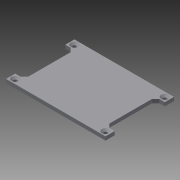
# Autodesk Inventor part: main body cover
Saved by Autodesk Inventor 2015 (Build 190159000, 159)
## iProperties
Created: 2019-05-11
Part Number: main body cover
Material: Generic
Document SubType Name: Modeling
Designer: Toby
Density: 1 g/cm^3
Appearance: Default
Author: Toby
Autodesk Inventor part; units mm, degrees
ref_plane "YZ Plane" through (0, 0, 0) normal (1, 0, 0) x (0, 1, 0)
ref_plane "XZ Plane" through (0, 0, 0) normal (0, 1, 0) x (-1, 0, 0)
ref_plane "XY Plane" through (0, 0, 0) normal (0, 0, 1) x (1, 0, 0)
sketch "Sketch1" plane through (0, 0, 0) normal (0, 0, 1) x (1, 0, 0)
  line L0 (-30.3644, 10.862) -> (24.0356, 10.862)
  line L1 (24.0356, 10.862) -> (24.0356, -26.538)
  line L2 (24.0356, -26.538) -> (-30.3644, -26.538)
  line L3 (-30.3644, -26.538) -> (-30.3644, 10.862)
  point P0 (0, 0)
  dimension "d0" = 54.4
  dimension "d1" = 37.4
  constraints: 8 end point, 2 parallel, 1 horizontal, 1 perpendicular
  measures "d0" distance of L0.start L0.end
  measures "d1" distance of L2.end L0.start
extrude "Extrusion1" add sketch "Sketch1" along normal blind 2
sketch "Sketch2" plane through (0, 0, 2) normal (0, 0, 1) x (1, 0, 0)
  line L0 (-30.3644, 10.862) -> (24.0356, 10.862) projected
  line L1 (-30.3644, 10.862) -> (-30.3644, -26.538) projected
  line L2 (-30.3644, -26.538) -> (24.0356, -26.538) projected
  line L3 (24.0356, -26.538) -> (24.0356, 10.862) projected
  point P0 (0, 0)
  point P1 (-27.8644, 8.362)
  point P2 (21.5356, -24.038)
  point P3 (21.5356, 8.362)
  point P4 (-27.8644, -24.038)
  dimension "d4" = 2.5
  dimension "d5" = 2.5
  dimension "d6" = 2.5
  dimension "d7" = 2.5
  measures "d4" distance from line of L0 point (-27.864, 8.362)
  measures "d5" distance from line of L1 point (-27.864, 8.362)
  measures "d6" distance from line of L2 point (21.536, -24.038)
  measures "d7" distance from line of L3 point (21.536, -24.038)
hole "Hole1" at (-27.8644, 8.362, 2) at (21.5356, -24.038, 2) at (21.5356, 8.362, 2) at (-27.8644, -24.038, 2) direction (0, 0, -1) diameter 2 depth 8 tip angle 118 countersink diameter 4 countersink angle 90
sketch "Sketch3" plane through (0, 0, 2) normal (0, 0, 1) x (1, 0, 0)
  line L0 (-30.3644, -26.538) -> (-30.3644, 10.862) projected
  line L1 (-30.3644, 5.862) -> (-25.3644, 5.862)
  line L2 (-25.3644, 5.862) -> (-25.3644, -21.538)
  line L3 (-25.3644, -21.538) -> (-30.3644, -21.538)
  line L4 (-30.3644, -21.538) -> (-30.3644, 5.862)
  line L5 (24.0356, 10.862) -> (24.0356, -26.538) projected
  line L6 (24.0356, 5.862) -> (19.0356, 5.862)
  line L7 (19.0356, 5.862) -> (19.0356, -21.538)
  line L8 (19.0356, -21.538) -> (24.0356, -21.538)
  line L9 (24.0356, -21.538) -> (24.0356, 5.862)
  line L10 (24.0356, 10.862) -> (-30.3644, 10.862) projected
  line L11 (-30.3644, -26.538) -> (24.0356, -26.538) projected
  point P0 (0, 0)
  dimension "d15" = 5
  dimension "d16" = 5
  dimension "d17" = 5
  dimension "d18" = 5
  constraints: 16 end point, 4 parallel, 4 point on line, 2 horizontal, 2 perpendicular
  measures "d15" distance between parallel lines of L10 L1
  measures "d16" distance between parallel lines of L11 L3
  measures "d17" distance between parallel lines of L0 L2
  measures "d18" distance between parallel lines of L5 L7
extrude "Extrusion2" cut sketch "Sketch3" against normal blind 2 contours L0 L1 L2 L3 | L8 L7 L6 L5
chamfer "Chamfer1" distance 2 angle 45 4 edges at (-25.3644, 5.862, 1) (-25.3644, -21.538, 1) (19.0356, -21.538, 1) (19.0356, 5.862, 1)
body "Solid1"
